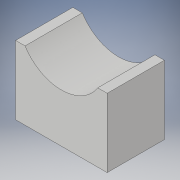
# Autodesk Inventor part: tankMount
Saved by Autodesk Inventor 2017 (Build 210142000, 142)
## iProperties
Created: 2016-04-26
Part Number: tankMount
Material: Generic
Document SubType Name: Modeling
Designer: kingb
Density: 1 g/cm^3
Appearance: Default
Author: kingb
Autodesk Inventor part; units mm, degrees
ref_plane "YZ Plane" through (0, 0, 0) normal (1, 0, 0) x (0, 1, 0)
ref_plane "XZ Plane" through (0, 0, 0) normal (0, 1, 0) x (-1, 0, 0)
ref_plane "XY Plane" through (0, 0, 0) normal (0, 0, 1) x (1, 0, 0)
sketch "Sketch1" plane through (0, 0, 0) normal (0, 0, 1) x (1, 0, 0)
  line L0 (0, 0) -> (203.2, 0)
  line L1 (203.2, 0) -> (203.2, 152.4)
  line L2 (0, 152.4) -> (0, 0)
  line L3 (203.2, 152.4) -> (196.85, 152.4)
  line L4 (6.35, 152.4) -> (0, 152.4)
  line L5 (101.6, 152.4) -> (101.6, 203.2)
  arc A0 (21.0275, 152.4) -> (182.1725, 152.4) centre (101.6, 203.2) ccw
  line L6 (6.35, 152.4) -> (21.0275, 152.4)
  line L7 (182.1725, 152.4) -> (196.85, 152.4)
  dimension "d0" = 203.2
  dimension "d1" = 152.4
  dimension "d5" = 50.8
  dimension "d6" = 190.5
  constraints: 16 end point, 3 horizontal, 3 parallel, 2 point on circle, 1 centre point, 1 coincident, 1 perpendicular, 1 vertical
  measures "d0" distance of L2.start L1.end
  measures "d1" distance of L1.end L0.end
  measures "d5" distance of L5.start L5.end
  measures "d6" diameter of A0
extrude "Extrusion1" add sketch "Sketch1" along normal blind 127
body "Solid1"
